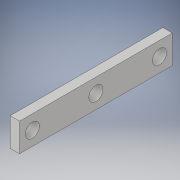
# Autodesk Inventor part: x 캐리지 벨트고정
Saved by Autodesk Inventor 2018 (Build 220112000, 112)
## iProperties
Created: 2019-01-22
Part Number: x 캐리지 벨트고정
Material: Generic
Document SubType Name: Modeling
Designer: User
Density: 1 g/cm^3
Appearance: Default
Author: User
Autodesk Inventor part; units mm, degrees
ref_plane "YZ Plane" through (0, 0, 0) normal (1, 0, 0) x (0, 1, 0)
ref_plane "XZ Plane" through (0, 0, 0) normal (0, 1, 0) x (-1, 0, 0)
ref_plane "XY Plane" through (0, 0, 0) normal (0, 0, 1) x (1, 0, 0)
sketch "스케치1" plane through (0, 0, 0) normal (1, 0, 0) x (0, 1, 0)
  line L0 (-6, 16.2) -> (-3, 16.2)
  line L1 (-3, 16.2) -> (0, 16.2)
  circle A0 centre (-3, 16.2) radius 1.5
  line L2 (-3, 16.2) -> (-3, 29.7)
  circle A1 centre (-3, 29.7) radius 1.5
  line L3 (-3, 16.2) -> (-3, 2.7)
  circle A2 centre (-3, 2.7) radius 1.5
  line L4 (-3, 29.7) -> (-3, 32.4)
  line L5 (-3, 32.4) -> (0, 32.4)
  line L6 (-3, 2.7) -> (-3, 0)
  line L7 (-3, 0) -> (0, 0)
  line L8 (0, 0) -> (0, 32.4)
  line L9 (-3, 32.4) -> (-6, 32.4)
  line L10 (-6, 0) -> (-3, 0)
  line L11 (-6, 0) -> (-6, 32.4)
  dimension "d0" = 3
  dimension "d1" = 3
  dimension "d2" = 3
  dimension "d3" = 13.5
  dimension "d4" = 3
  dimension "d5" = 13.5
  dimension "d6" = 3
  dimension "d7" = 2.7
  dimension "d8" = 2.7
  constraints: 24 end point, 5 vertical, 4 coincident, 3 centre point, 3 horizontal, 2 perpendicular, 1 parallel, 1 point on line
  measures "d0" distance of L0.start L0.end
  measures "d1" distance of L0.end L1.end
  measures "d2" diameter of A0
  measures "d3" distance of L3.start L2.end
  measures "d4" diameter of A1
  measures "d5" distance of L3.start L3.end
  measures "d6" diameter of A2
  measures "d7" distance of L4.start L4.end
  measures "d8" distance of L6.start L7.start
extrude "돌출1" add sketch "스케치1" along normal blind 2.5 contours L11 L9 L4 A1 L2 A0 L0 | L0 A0 L3 A2 L6 L10 L11 | L2 A1 L4 L5 L8 L1 A0 | A0 L1 L8 L7 L6 A2 L3
chamfer "모따기1" distance 0.5 angle 45 4 edges at (0, 0, 16.2) (0, -1.5, 0) (0, -6, 16.2) (0, -4.5, 32.4)
